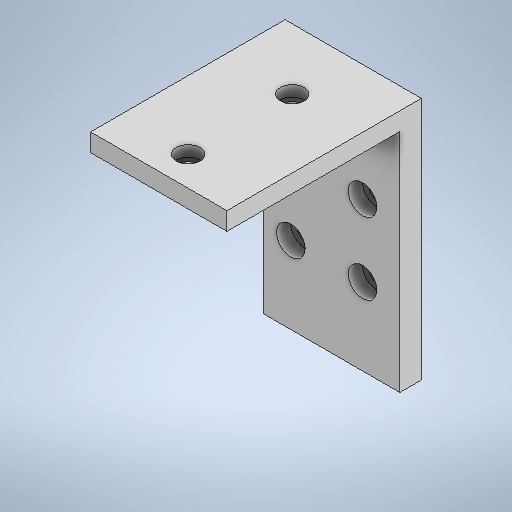
# Autodesk Inventor part: TS_Adapter_Greifer_int
Saved by Autodesk Inventor 2025.2 (Build 292293000, 293)
## iProperties
Created: 2025-06-16
Part Number: TS_Adapter_Greifer_int
Material: Generisch
Document SubType Name: Modeling
Designer: tino
Density: 1 g/cm^3
Appearance: Vorgabe
Author: tino
Autodesk Inventor part; units mm, degrees
ref_plane "YZ Plane" through (0, 0, 0) normal (1, 0, 0) x (0, 1, 0)
ref_plane "XZ Plane" through (0, 0, 0) normal (0, 1, 0) x (-1, 0, 0)
ref_plane "XY Plane" through (0, 0, 0) normal (0, 0, 1) x (1, 0, 0)
sketch "Skizze1" plane through (0, 0, 0) normal (0, 0, 1) x (1, 0, 0)
  line L0 (-19, 27.1) -> (19, 27.1)
  line L1 (19, 27.1) -> (19, -27.1)
  line L2 (19, -27.1) -> (-19, -27.1)
  line L3 (-19, -27.1) -> (-19, 27.1)
  line L4 (0, 37.94) -> (0, -37.94) projected
  line L5 (-26.6, 0) -> (26.6, 0) projected
  point P0 (0, 0)
  dimension "d0" = 38
  dimension "d1" = 54.2
  dimension "d46" = 19
  dimension "d47" = 27.1
  constraints: 8 end point, 2 parallel, 1 horizontal, 1 perpendicular
  measures "d0" distance of L1.end L2.end
  measures "d1" distance of L2.end L0.start
  measures "d46" distance between parallel lines of L3 L4
  measures "d47" distance between parallel lines of L5 L2
extrude "Extrusion1" add sketch "Skizze1" along normal blind 63
sketch "Skizze2" plane through (0, 0, 63) normal (0, 0, 1) x (1, 0, 0)
  line L0 (-19, -27.1) -> (19, -27.1) projected
  line L1 (-19, -27.1) -> (19, -27.1)
  line L2 (19, -27.1) -> (19, 21.1)
  line L3 (19, 21.1) -> (-19, 21.1)
  line L4 (-19, 21.1) -> (-19, -27.1)
  line L5 (-19, 27.1) -> (-19, -27.1) projected
  line L6 (19, 27.1) -> (-19, 27.1) projected
  point P0 (0, 0)
  dimension "d4" = 38
  dimension "d6" = 6
  constraints: 8 end point, 2 parallel, 1 collinear, 1 horizontal, 1 perpendicular, 1 point on line
  measures "d4" distance of L2.end L3.end
  measures "d6" distance between parallel lines of L6 L3
extrude "Extrusion2" cut sketch "Skizze2" against normal through all
sketch "Skizze6" plane through (-19, 27.1, 0) normal (0, 1, 0) x (1, 0, 0)
  line L0 (38, -63) -> (0, -63) projected
  line L1 (38, 0) -> (0, 0) projected
  line L2 (19, 12.6) -> (19, -75.6) projected
  point P0 (19, 0)
  point P1 (19, -44)
  point P2 (19, -19)
  dimension "d48" = 25
  dimension "d49" = 63
  dimension "d50" = 19
  constraints: 1 point on line, 1 vertical alignment
  measures "d48" distance of point (19, -19) point (19, -44)
  measures "d49" distance between parallel lines of L0 L1
  measures "d50" distance from line of L1 point (19, -19)
hole "Bohrung4" at (0, 27.1, 44) at (0, 27.1, 19) direction (0, -1, 0) diameter 5 depth 2.5
sketch "Skizze13" plane through (-19, 21.1, 63) normal (0, -1, 0) x (1, 0, 0)
  line L0 (38, 0) -> (38, -63) projected
  line L1 (0, -63) -> (0, 0) projected
  line L2 (38, -63) -> (0, -63) projected
  line L3 (0, 0) -> (38, 0) projected
  point P0 (19, -63)
  point P1 (7.6, -21.5)
  point P2 (27.6, -21.5)
  point P3 (27.6, -41.5)
  point P4 (7.6, -41.5)
  dimension "d102" = 20
  dimension "d103" = 20
  dimension "d104" = 38
  dimension "d105" = 7.6
  dimension "d106" = 63
  dimension "d107" = 21.5
  constraints: 2 horizontal alignment, 2 vertical alignment
  measures "d102" distance of point (27.6, -21.5) point (7.6, -21.5)
  measures "d103" distance of point (27.6, -21.5) point (27.6, -41.5)
  measures "d104" distance between parallel lines of L0 L1
  measures "d105" distance from line of L1 point (7.6, -41.5)
  measures "d106" distance between parallel lines of L2 L3
  measures "d107" distance from line of L2 point (27.6, -41.5)
hole "Bohrung6" at (-11.4, 21.1, 41.5) at (8.6, 21.1, 41.5) at (8.6, 21.1, 21.5) at (-11.4, 21.1, 21.5) direction (0, 1, 0) diameter 4.5 end through all counterbore diameter 8 counterbore depth 4 clearance for "Innensechskantkopfschraube" size "M4" standard "ANSI Metrisches M Profil"
sketch "Skizze14" plane through (0, 0, 63) normal (0, 0, 1) x (1, 0, 0)
  line L0 (19, 27.1) -> (-19, 27.1) projected
  line L1 (-19, 27.1) -> (19, 27.1)
  line L2 (19, 27.1) -> (19, -27.1)
  line L3 (19, -27.1) -> (-19, -27.1)
  line L4 (-19, -27.1) -> (-19, 27.1)
  line L5 (19, 21.1) -> (19, 27.1) projected
  point P0 (0, 0)
  dimension "d115" = 54.2
  constraints: 8 end point, 2 parallel, 1 collinear, 1 horizontal, 1 perpendicular
  measures "d115" distance between parallel lines of L0 L3
extrude "Extrusion8" add sketch "Skizze14" along normal blind 5
sketch "Skizze15" plane through (0, 0, 68) normal (0, 0, -1) x (-1, 0, 0)
  line L0 (-19, 21.1) -> (19, 21.1) projected
  point P0 (0, 0)
  point P1 (0, 10.1)
  point P2 (0, -18.9)
  dimension "d118" = 11
  dimension "d119" = 29
  constraints: 2 vertical alignment
  measures "d118" distance from line of point (0, 10.1) L0
  measures "d119" distance of point (0, -18.9) point (0, 10.1)
hole "Bohrung7" at (0, 10.1, 68) at (0, -18.9, 68) direction (0, 0, -1) diameter 6.6 end through all clearance for "Innensechskantkopfschraube" size "M6" standard "ANSI Metrisches M Profil"
sketch "Skizze16" plane through (0, 0, 63) normal (0, 0, -1) x (-1, 0, 0)
  circle A0 centre (0, -18.9) radius 5.5 projected
  circle A1 centre (0, -18.9) radius 3.3 projected
  circle A2 centre (0, -18.9) radius 3.3 projected
  circle A3 centre (0, 10.1) radius 3.3 projected
  line L0 (19, 21.1) -> (-19, 21.1) projected
  line L1 (-19, -27.1) -> (-19, 21.1) projected
  line L2 (19, -27.1) -> (-19, -27.1) projected
  line L3 (19, 21.1) -> (19, -27.1) projected
  circle A4 centre (0, 10.1) radius 5.5 projected
  circle A5 centre (0, 10.1) radius 3.3 projected
  point P0 (0, 0)
  constraints: 2 coincident
hole "Bohrung8" at (0, 10.1, 63) at (0, -18.9, 63) direction (0, 0, 1) diameter 9 depth 2
equation "\"d46\" = 0.5 * d0"
equation "\"d47\" = 0.5 * d1"
equation "\"d50\" = -0.5 * d48 + 0.5 * d49"
equation "\"d107\" = -0.5 * d103 + 0.5 * d106"
